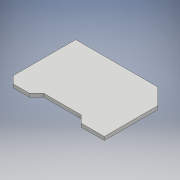
# Autodesk Inventor part: Game_TurmoilPolicy
Saved by Autodesk Inventor 2018 (Build 220112000, 112)
## iProperties
Created: 2021-04-21
Part Number: Game_TurmoilPolicy
Material: Generic
Document SubType Name: Modeling
Designer: Bradley
Density: 1 g/cm^3
Appearance: Default
Author: Bradley
Autodesk Inventor part; units mm, degrees
ref_plane "YZ Plane" through (0, 0, 0) normal (1, 0, 0) x (0, 1, 0)
ref_plane "XZ Plane" through (0, 0, 0) normal (0, 1, 0) x (-1, 0, 0)
ref_plane "XY Plane" through (0, 0, 0) normal (0, 0, 1) x (1, 0, 0)
sketch "Sketch1" plane through (0, 0, 0) normal (0, 0, 1) x (1, 0, 0)
  line L0 (-23.5, -19.5) -> (27.5, -19.5)
  line L1 (27.5, -19.5) -> (27.5, 10.5)
  line L2 (18.5, 19.5) -> (-27.5, 19.5)
  line L3 (-27.5, 19.5) -> (-27.5, -15.5)
  line L4 (-27.5, -19.5) -> (27.5, 19.5) construction
  line L5 (27.5, -19.5) -> (-27.5, 19.5) construction
  line L6 (18.5, 19.5) -> (27.5, 10.5)
  line L7 (-27.5, -15.5) -> (-23.5, -19.5)
  line L8 (-14.5, -19.5) -> (-10.5, -15.5)
  line L9 (-10.5, -15.5) -> (10.5, -15.5)
  line L10 (10.5, -15.5) -> (14.5, -19.5)
  point P0 (0, 0)
  dimension "d0" = 55
  dimension "d1" = 39
  dimension "d2" = 9
  dimension "d3" = 9
  dimension "d4" = 4
  dimension "d5" = 4
  dimension "d11" = 17
  dimension "d12" = 17
  constraints: 22 end point, 7 point on line, 3 perpendicular, 2 horizontal, 2 midpoint, 2 parallel
  measures "d0" distance of L2.end L4.end
  measures "d1" distance of L4.end L0.end
  measures "d2" distance of L2.start L4.end
  measures "d3" distance of L1.end L4.end
  measures "d4" distance of L3.end L4.start
  measures "d5" distance of L0.start L4.start
  measures "d11" distance from line of L3 L8.end
  measures "d12" distance from line of L1 L9.end
extrude "Extrusion1" add sketch "Sketch1" along normal mid plane 1.91 contours L7 L3 L2 L6 L1 L0 L10 L9 L8
equation "\"d3\" = d2"
equation "\"d4\" = d5"
equation "\"d12\" = d11"
body "Solid1"
